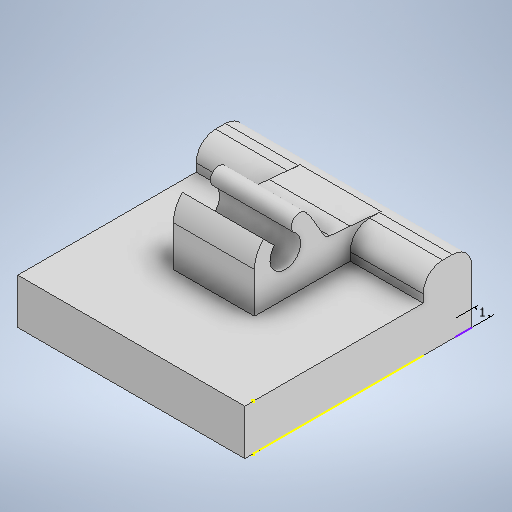
# Autodesk Inventor part: Part1
Saved by Autodesk Inventor 2025.2 (Build 292293000, 293)
## iProperties
Created: 2025-02-01
Part Number: Part1
Material: Generic
Document SubType Name: Modeling
Designer: Kuba
Density: 1 g/cm^3
Appearance: Default
Author: Kuba
## iProperties of the stored document Part1_3DPrint.ipt
Created: 2025-02-01
Part Number: Part1_3DPrint
Material: Generic
Document SubType Name: Modeling
Designer: Kuba
Density: 1 g/cm^3
Appearance: Default
Author: Kuba
Autodesk Inventor part; units mm, degrees
ref_plane "YZ Plane" through (0, 0, 0) normal (1, 0, 0) x (0, 1, 0)
ref_plane "XZ Plane" through (0, 0, 0) normal (0, 1, 0) x (-1, 0, 0)
ref_plane "XY Plane" through (0, 0, 0) normal (0, 0, 1) x (1, 0, 0)
sketch "Sketch1" plane through (0, 0, 0) normal (0, 1, 0) x (-1, 0, 0)
  line L0 (0, 0) -> (14, 0)
  line L1 (14, 0) -> (14, -13.5)
  line L2 (14, -13.5) -> (0, -13.5)
  line L3 (0, -13.5) -> (0, 0)
  dimension "d0" = 14
  dimension "d1" = 13.5
  constraints: 8 end point, 2 parallel, 1 horizontal, 1 perpendicular
  measures "d0" distance of L1.end L2.end
  measures "d1" distance of L0.end L1.end
extrude "Extrusion1" add sketch "Sketch1" along normal blind 2.8
sketch "Sketch2" plane through (0, 2.8, 0) normal (0, 1, 0) x (1, 0, 0)
  point P0 (0, 0)
sketch "Sketch3" plane through (0, 2.8, 0) normal (0, 1, 0) x (1, 0, 0)
  line L0 (0, 13.5) -> (-14, 13.5) projected
  line L1 (-14, 13.5) -> (-14, 10.5)
  line L2 (-14, 13.5) -> (-14, 0) projected
  line L3 (-14, 10.5) -> (0, 10.5)
  line L4 (0, 10.5) -> (0, 13.5)
  line L5 (0, 13.5) -> (-14, 13.5)
  line L6 (-14, 13.5) -> (-14, 10.5)
  point P0 (0, 0)
  dimension "d4" = 3
  constraints: 10 end point, 2 parallel, 1 horizontal, 1 perpendicular, 1 point on line
  measures "d4" distance of L0.end L1.end
extrude "Extrusion2" add sketch "Sketch3" along normal blind 1.7
fillet "Fillet1" radius 1.2 1 edges at (-7, 4.5, -13.5)
fillet "Fillet2" radius 1.2 1 edges at (-7, 4.5, -10.5)
sketch "Sketch4" plane through (0, 0, 0) normal (0, -1, 0) x (1, 0, 0)
  line L0 (0, -13.5) -> (-14, -13.5) projected
  line L1 (0, -13.5) -> (-1, -13.5)
  line L2 (-14, -13.5) -> (-14, 0) projected
  line L3 (-14, 0) -> (0, 0) projected
  line L4 (0, 0) -> (0, -10.5) projected
  line L5 (0, -13.5) -> (-1, -13.5)
  line L6 (0, -12.5) -> (0, -13.5)
  line L7 (-14, 0) -> (-13, 0)
  line L8 (-14, -1) -> (-14, 0)
  dimension "d9" = 1
  constraints: 10 end point, 2 horizontal, 1 point on line
  measures "d9" distance of L0.start L1.end
sketch "Sketch5" plane through (0, 0, 0) normal (0, -1, 0) x (1, 0, 0)
  point P0 (0, 0)
sketch "Sketch6" plane through (0, 0, 0) normal (0, -1, 0) x (1, 0, 0)
  line L0 (-14, -13.5) -> (-14, -12.3) projected
  line L1 (-14, -13.5) -> (-14, 0.5)
  line L2 (-14, 0.5) -> (0, 0.5)
  line L3 (0, 0.5) -> (0, 0)
  line L4 (0, 0) -> (-14, 0)
  line L5 (-14, 0) -> (-14, 0.5)
  dimension "d15" = 14
  constraints: 10 end point, 2 parallel, 1 collinear, 1 horizontal, 1 perpendicular
  measures "d15" distance of L0.start L1.end
extrude "Extrusion3" add sketch "Sketch6" against normal blind 2.8
sketch "Sketch7" plane through (0, 0, 0) normal (0, -1, 0) x (1, 0, 0)
  line L0 (-14, -13.5) -> (-14, -12.3) projected
  line L1 (-14, -13.5) -> (-13, -13.5)
  line L2 (-14, -12.5) -> (-14, -13.5)
  line L3 (0, -13.5) -> (0, 0.5) projected
  line L4 (0, 0.5) -> (-1, 0.5)
  line L5 (0, -0.5) -> (0, 0.5)
  line L6 (-14, -13.5) -> (-14, 0.5) projected
  line L7 (-14, 0.5) -> (-13, 0.5)
  line L8 (-14, -0.5) -> (-14, 0.5)
  line L9 (0, -13.5) -> (-14, -13.5) projected
  line L10 (0, -13.5) -> (-1, -13.5)
  line L11 (0, -12.5) -> (0, -13.5)
  line L12 (-14, -13.5) -> (-7, -13.5)
  line L13 (-7, -13.5) -> (-7, 0.5)
  line L14 (-7, 0.5) -> (-7.707, 0.5)
  line L15 (-14, 0.5) -> (0, 0.5) projected
  line L16 (-7, 0.5) -> (-6.293, 0.5)
  line L17 (-7.707, 0.5) -> (-14, -5.793)
  line L18 (-6.293, 0.5) -> (-14, -7.207)
  line L19 (-7.707, 0.5) -> (0, -7.207)
  line L20 (-6.293, 0.5) -> (0, -5.793)
  line L21 (-6.293, -13.5) -> (0, -7.207)
  line L22 (-7.707, -13.5) -> (0, -5.793)
  line L23 (-7.707, -13.5) -> (-14, -7.207)
  line L24 (-6.293, -13.5) -> (-14, -5.793)
  line L25 (-14, -13.5) -> (-13.293, -13.5)
  line L26 (-13.293, -13.5) -> (-14, -13.5)
  line L27 (-14, -13.5) -> (-14, -12.793)
  line L28 (-14, -12.793) -> (-13.293, -12.793)
  line L29 (-13.293, -12.793) -> (-13.293, -13.5)
  line L30 (0, 0.5) -> (-0.707, 0.5)
  line L31 (-0.707, 0.5) -> (-0.707, -0.207)
  line L32 (-0.707, -0.207) -> (0, -0.207)
  line L33 (0, -0.207) -> (0, 0.5)
  line L34 (-13.293, -13.5) -> (0, -0.207)
  line L35 (-0.707, 0.5) -> (-14, -12.793)
  line L36 (0, -13.5) -> (-0.707, -13.5)
  line L37 (-0.707, -13.5) -> (-0.707, -12.793)
  line L38 (-0.707, -12.793) -> (0, -12.793)
  line L39 (0, -12.793) -> (0, -13.5)
  line L40 (-14, 0.5) -> (-13.293, 0.5)
  line L41 (-13.293, 0.5) -> (-13.293, -0.207)
  line L42 (-13.293, -0.207) -> (-14, -0.207)
  line L43 (-14, -0.207) -> (-14, 0.5)
  line L44 (-14, -0.207) -> (-0.707, -13.5)
  line L45 (0, -12.793) -> (-13.293, 0.5)
  line L46 (-13.293, -12.793) -> (-0.707, -12.793)
  line L47 (-0.707, -12.793) -> (-0.707, -0.207)
  line L48 (-0.707, -0.207) -> (-13.293, -0.207)
  line L49 (-13.293, -0.207) -> (-13.293, -12.793)
  point P0 (0, 0)
  point P1 (-1.414, -0.207)
  point P2 (-5.586, -0.207)
  point P3 (-3.5, -2.293)
  point P4 (-0.707, -5.086)
  point P5 (-0.707, -0.914)
  point P6 (-2.793, -3)
  point P7 (-6.293, -6.5)
  point P8 (-3.5, -9.293)
  point P9 (-0.707, -6.5)
  point P10 (-3.5, -3.707)
  point P11 (-0.707, -12.086)
  point P12 (-0.707, -7.914)
  point P13 (-2.793, -10)
  point P14 (-5.586, -12.793)
  point P15 (-1.414, -12.793)
  point P16 (-3.5, -10.707)
  point P17 (-7, -7.207)
  point P18 (-9.793, -10)
  point P19 (-7, -12.793)
  point P20 (-4.207, -10)
  point P21 (-9.793, -3)
  point P22 (-7, -5.793)
  point P23 (-4.207, -3)
  point P24 (-7, -0.207)
  point P25 (-8.414, -0.207)
  point P26 (-12.586, -0.207)
  point P27 (-10.5, -2.293)
  point P28 (-13.293, -0.914)
  point P29 (-13.293, -5.086)
  point P30 (-11.207, -3)
  point P31 (-7.707, -6.5)
  point P32 (-10.5, -3.707)
  point P33 (-13.293, -6.5)
  point P34 (-10.5, -9.293)
  point P35 (-13.293, -7.914)
  point P36 (-13.293, -12.086)
  point P37 (-11.207, -10)
  point P38 (-12.586, -12.793)
  point P39 (-8.414, -12.793)
  point P40 (-10.5, -10.707)
  dimension "d26" = 7
  dimension "d27" = 0.707
  dimension "d28" = 0.707
  dimension "d30" = 0.707
  dimension "d31" = 0.707
  dimension "d32" = 0.707
  dimension "d33" = 0.707
  dimension "d34" = 0.707
  constraints: 90 end point, 14 parallel, 10 point on line, 9 horizontal, 9 perpendicular, 1 midpoint
  measures "d26" distance of L0.start L12.end
  measures "d27" distance of L13.end L14.end
  measures "d28" distance of L13.end L16.end
  measures "d30" distance of L26.end L27.end
  measures "d31" distance of L32.end L31.end
  measures "d32" distance of L31.end L30.end
  measures "d33" distance of L37.end L38.end
  measures "d34" distance of L41.end L42.end
extrude "Extrusion4" cut sketch "Sketch7" against normal blind 1 contours L49 L23 L35 | L34 L23 L46 | L24 L18 L44 L35 | L24 L34 L13 | L13 L44 L22 | L49 L44 L17 | L21 L44 L46 | L45 L18 L13 | L13 L19 L35 | L34 L19 L22 L45 | L45 L48 L17 | L21 L47 L45 | L48 L35 L20 | L34 L47 L20
sketch "Sketch8" plane through (0, 2.8, 0) normal (0, 1, 0) x (1, 0, 0)
  point P0 (0, 0)
sketch "Sketch9" plane through (0, 2.8, 0) normal (0, 1, 0) x (1, 0, 0)
  line L0 (-14, 13.5) -> (-14, -0.5) projected
  line L1 (-14, -0.5) -> (0, -0.5)
  line L2 (-14, -0.5) -> (-9.5, -0.5)
  line L3 (0, 13.5) -> (0, -0.5) projected
  line L4 (0, -0.5) -> (-4.5, -0.5)
  line L5 (-9.5, -0.5) -> (-9.5, 13.5)
  line L6 (-4.5, -0.5) -> (-4.5, 13.5)
  line L7 (-9.5, -0.5) -> (-4.5, -0.5)
  line L8 (-4.5, -0.5) -> (-4.5, 4)
  line L9 (-4.5, 4) -> (-9.5, 4)
  line L10 (-9.5, 4) -> (-9.5, -0.5)
  line L11 (-9.5, 13.5) -> (-4.5, 13.5)
  line L12 (-4.5, 13.5) -> (-4.5, 4)
  line L13 (-4.5, 4) -> (-9.5, 4)
  line L14 (-9.5, 4) -> (-9.5, 13.5)
  line L15 (-9.5, 4) -> (-4.5, 4)
  line L16 (-4.5, 4) -> (-4.5, 9)
  line L17 (-4.5, 9) -> (-9.5, 9)
  line L18 (-9.5, 9) -> (-9.5, 4)
  line L19 (-9.5, 13.5) -> (-4.5, 13.5)
  line L20 (-4.5, 13.5) -> (-4.5, 9)
  line L21 (-4.5, 9) -> (-9.5, 9)
  line L22 (-9.5, 9) -> (-9.5, 13.5)
  point P0 (0, 0)
  dimension "d37" = 4.5
  dimension "d38" = 4.5
  dimension "d39" = 4.5
  dimension "d40" = 5
  constraints: 42 end point, 8 parallel, 5 horizontal, 4 perpendicular, 4 point on line, 2 vertical
  measures "d37" distance of L0.end L2.end
  measures "d38" distance of L1.end L4.end
  measures "d39" distance of L8.end L7.end
  measures "d40" distance of L16.end L15.end
extrude "Extrusion5" add sketch "Sketch9" along normal blind 5 contours L5 L17 L6 L9
extrude "Extrusion6" add sketch "Sketch9" along normal blind 2 contours L5 L11 L6 L17
sketch "Sketch10" plane through (-9.5, 2.8, -10.5) normal (-1, 0, 0) x (0, 0, 1)
  line L0 (1.5, 2) -> (1.5, 5) projected
  line L1 (1.5, 2) -> (-1.9069, 1.6952)
  arc A0 (-1.8, 1.7) -> (-3, 0.5) centre (-1.8, 0.5) ccw projected
  line L2 (-3, 0.5) -> (-3, 2) projected
  line L3 (1.5, 2) -> (-3, 2)
  line L4 (-3, 2) -> (-3, 0.5)
  line L5 (-3, 2) -> (-3, 0.5)
  line L6 (-3, 0.5) -> (-1.9069, 1.6952)
  point P0 (10.5, -2.8)
  constraints: 10 end point, 2 collinear, 2 tangent, 1 horizontal, 1 point on circle
extrude "Extrusion7" cut sketch "Sketch10" against normal through all contours L1 A0 L2 L3
sketch "Sketch11" plane through (-9.5, 2.8, -10.5) normal (-1, 0, 0) x (0, 0, 1)
  line L0 (1.5, 5) -> (4, 5)
  line L1 (1.5, 5) -> (6.5, 5) projected
  line L2 (4, 5) -> (4, 0)
  line L3 (0, 0) -> (6.5, 0) projected
  circle A0 centre (4, 2.5) radius 0.95
  line L4 (4.95, 2.5) -> (5.9, 2.5)
  line L5 (3.05, 2.5) -> (2.1, 2.5)
  circle A1 centre (4, 2.5) radius 1.9
  line L6 (5.9, 2.5) -> (5.9, 0)
  line L7 (2.1, 2.5) -> (2.1, 0)
  line L8 (4, 2.5) -> (4.6718, 3.1718)
  line L9 (4, 2.5) -> (4.95, 2.5) construction
  line L10 (4.6718, 3.1718) -> (5.3435, 3.8435)
  line L11 (4, 2.5) -> (2.8317, 4.5236)
  line L12 (4, 2.5) -> (6.3367, 2.5) construction
  line L13 (3.05, 4.1454) -> (3.525, 3.3227)
  line L14 (3.05, 4.1454) -> (3.2875, 3.7341)
  line L15 (3.2875, 3.7341) -> (3.1143, 3.6341)
  circle A2 centre (3.1143, 3.6341) radius 0.5154
  line L16 (1.5, 1.9745) -> (2.3558, 3.4522)
  line L17 (1.5, 1.9745) -> (1.5, 5)
  line L18 (1.5, 5) -> (6.5, 5)
  line L19 (6.5, 0) -> (6.5, 5) projected
  line L20 (6.5, 0) -> (5.9, 0)
  point P0 (10.5, -2.8)
  point P1 (2.6337, 3.8204)
  point P2 (3.05, 4.1454)
  point P3 (4, 4.4)
  point P4 (4, 3.45)
  dimension "d47" = 1.9
  dimension "d48" = 0.95
  dimension "d49" = 0.95
  dimension "d50" = 45
  dimension "d51" = 120
  dimension "d52" = 0.475
  dimension "d53" = 0.2
  constraints: 36 end point, 8 point on circle, 5 perpendicular, 5 point on line, 3 horizontal, 3 midpoint, 3 tangent, 2 centre point, 2 coincident, 2 collinear, 2 equal length, 3 other
  measures "d47" diameter of A0
  measures "d48" distance of L4.start L4.end
  measures "d49" distance of L5.start L5.end
  measures "d50" angle of L9 L8
  measures "d51" angle of L12 L11
  measures "d52" distance of L13.start L14.end
  measures "d53" distance of L14.end L15.end
extrude "Extrusion8" cut sketch "Sketch11" against normal through all contours L0 L2 A1 A2 L16 L17
extrude "Extrusion9" cut sketch "Sketch11" against normal through all contours L1 L19 L3 L6 A1 L2
extrude "Extrusion10" cut sketch "Sketch11" against normal through all contours A0 L8 L2 | L2 L11 A0 | L8 A0 L2 | L2 A0 A2 L11 | A2 A0
extrude "Extrusion11" cut sketch "Sketch11" against normal through all contours L2 A0 A2 A1
extrude "Extrusion12" cut sketch "Sketch11" against normal through all contours A1 L10 A0 L2
sketch "Sketch12" plane through (-9.5, 2.8, -10.5) normal (-1, 0, 0) x (0, 0, 1)
  point P0 (10.5, -2.8)
sketch "Sketch13" plane through (-9.5, 2.8, -10.5) normal (-1, 0, 0) x (0, 0, 1)
  line L0 (0, 1.8659) -> (1.8124, 2.028)
  line L1 (1.5, 2) -> (-1.9069, 1.6952) projected
  line L2 (1.8124, 2.028) -> (1.8124, 0)
  line L3 (5.9, 0) -> (0, 0) projected
  line L4 (0, 0) -> (0, 1.8659)
  line L5 (1.8124, 0) -> (0, 0)
  point P0 (10.5, -2.8)
  point P1 (-1.9069, 1.6952)
  constraints: 6 end point, 1 parallel, 1 perpendicular, 1 point on line, 1 vertical, 4 other
extrude "Extrusion13" add sketch "Sketch13" against normal blind 5
fillet "Fillet3" radius 0.5 1 edges at (-7, 4.8015, -8.9844)
body "Solid1"
